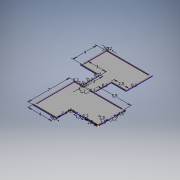
# Autodesk Inventor part: floormap
Saved by Autodesk Inventor 2019.4 (Build 234330000, 330)
## iProperties
Part Number: floormap
Material: Generic
Document SubType Name: Modeling
Designer: Jorge
Appearance: Default
Author: Jorge
Autodesk Inventor part; units mm, degrees
ref_plane "YZ Plane" through (0, 0, 0) normal (1, 0, 0) x (0, 1, 0)
ref_plane "XZ Plane" through (0, 0, 0) normal (0, 1, 0) x (-1, 0, 0)
ref_plane "XY Plane" through (0, 0, 0) normal (0, 0, 1) x (1, 0, 0)
sketch "Sketch1" plane through (0, 0, 0) normal (0, 1, 0) x (-1, 0, 0)
  line L0 (200, -200) -> (200, -1700)
  line L1 (200, -200) -> (2200, -200)
  line L2 (2200, -200) -> (2200, 0)
  line L3 (2200, 0) -> (0, 0)
  line L4 (0, 0) -> (0, -1700)
  line L5 (0, -1700) -> (200, -1700)
  line L6 (0, -1700) -> (0, -2900) construction
  line L7 (0, -2900) -> (200, -2900)
  line L8 (200, -2900) -> (200, -1700) construction
  line L9 (200, -2900) -> (200, -4400)
  line L10 (200, -4400) -> (5700, -4400)
  line L11 (5700, -4400) -> (5700, -4600)
  line L12 (5700, -4600) -> (5400, -4600)
  line L13 (0, -4600) -> (0, -2900)
  line L14 (200, -1700) -> (1400, -1700) construction
  line L15 (5700, -4400) -> (6900, -4400) construction
  line L16 (6900, -4400) -> (6900, -4600)
  line L17 (6900, -4600) -> (5700, -4600) construction
  line L18 (2200, -200) -> (3700, -200) construction
  line L19 (3700, -200) -> (3700, 0)
  line L20 (3700, 0) -> (2200, 0) construction
  line L21 (6900, -4600) -> (7200, -4600)
  line L22 (8400, -4400) -> (6900, -4400)
  line L23 (8400, -4600) -> (8600, -4600)
  line L24 (8600, -4600) -> (8600, 2400)
  line L25 (8600, 2400) -> (4600, 2400)
  line L26 (4600, 2400) -> (4600, 0)
  line L27 (4600, 0) -> (3700, 0)
  line L28 (3700, -200) -> (4800, -200)
  line L29 (4800, -200) -> (4800, 2200)
  line L30 (4800, 2200) -> (8400, 2200)
  line L31 (8400, 2200) -> (8400, -4400)
  line L32 (7200, -4600) -> (7200, -7600)
  line L33 (7200, -7600) -> (10200, -7600)
  line L34 (10200, -7600) -> (10200, -11600)
  line L35 (5200, -4600) -> (5200, -7400)
  line L36 (10400, -11800) -> (10400, -7400)
  line L37 (10400, -7400) -> (7400, -7400)
  line L38 (7400, -7400) -> (7400, -4600)
  line L39 (2700, -11800) -> (2700, -7400)
  line L40 (2700, -7400) -> (5200, -7400)
  line L41 (5400, -7600) -> (2900, -7600)
  line L42 (5400, -7600) -> (5400, -4600)
  line L43 (5200, -4600) -> (0, -4600)
  line L44 (7400, -4600) -> (8400, -4600)
  line L45 (10200, -11600) -> (2900, -11600)
  line L46 (2700, -11800) -> (10400, -11800)
  line L47 (2900, -7600) -> (2900, -11600)
  line L48 (0, -1700) -> (0, -2900)
  line L49 (2200, 0) -> (3700, 0)
  dimension "d1" = 1500
  dimension "d2" = 2000
  dimension "d3" = 200
  dimension "d4" = 2200
  dimension "d5" = 1200
  dimension "d6" = 1500
  dimension "d7" = 5500
  dimension "d8" = 200
  dimension "d9" = 1200
  dimension "d10" = 1200
  dimension "d11" = 1500
  dimension "d12" = 1500
  dimension "d14" = 7000
  dimension "d15" = 4000
  dimension "d16" = 1100
  dimension "d17" = 2400
  dimension "d18" = 3000
  dimension "d19" = 3000
  dimension "d20" = 4000
  dimension "d22" = 300
  dimension "d23" = 200
  dimension "d25" = 200
  dimension "d27" = 200
  dimension "d29" = 300
  dimension "d30" = 200
  dimension "d32" = 200
  dimension "d33" = 200
  dimension "d34" = 200
  dimension "d35" = 2500
  dimension "d36" = 200
  constraints: 100 end point, 27 perpendicular, 9 horizontal, 7 vertical, 6 collinear, 6 parallel, 3 point on line, 2 coincident, 2 other
  measures "d1" distance of L0.start L0.end
  measures "d2" distance of L0.start L1.end
  measures "d3" distance of L1.end L2.end
  measures "d4" distance of L2.end L3.end
  measures "d5" distance of L4.end L6.end
  measures "d6" distance of L7.end L9.end
  measures "d7" distance of L9.end L10.end
  measures "d8" distance of L10.end L11.end
  measures "d9" distance of L0.end L14.end
  measures "d10" distance of L10.end L15.end
  measures "d11" distance of L1.end L18.end
  measures "d12" distance of L16.end L23.start
  measures "d14" distance of L23.end L24.end
  measures "d15" distance of L24.end L25.end
  measures "d16" distance of L18.end L28.end
  measures "d17" distance of L28.end L29.end
  measures "d18" distance of L21.end L32.end
  measures "d19" distance of L32.end L33.end
  measures "d20" distance of L33.end L34.end
  measures "d22" distance between parallel lines of L16 L32
  measures "d23" distance between parallel lines of L38 L32
  measures "d25" distance between parallel lines of L33 L37
  measures "d27" distance between parallel lines of L36 L34
  measures "d29" distance between parallel lines of L11 L42
  measures "d30" distance between parallel lines of L42 L35
  measures "d32" distance between parallel lines of L31 L24
  measures "d33" distance between parallel lines of L46 L45
  measures "d34" distance between parallel lines of L47 L39
  measures "d35" distance between parallel lines of L47 L42
  measures "d36" distance between parallel lines of L29 L26
extrude "Extrusion1" add sketch "Sketch1" along normal blind 200 contours L0 L5 L4 L3 L2 L1 | L7 L9 L10 L11 L12 L42 L41 L47 L45 L34 L33 L32 L21 L16 L22 L31 L30 L29 L28 L19 L27 L26 L25 L24 L23 L44 L38 L37 L36 L46 L39 L40 L35 L43 L13
extrude "Extrusion2" add sketch "Sketch1" against normal blind 100
body "Solid1"
